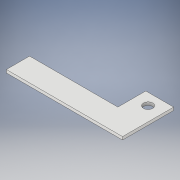
# Autodesk Inventor part: Y-axis X-axis Flag
Saved by Autodesk Inventor 2018 (Build 220112000, 112)
## iProperties
Created: 2013-10-27
Part Number: Y-axis X-axis Flag
Material: Nylon 6/6
Document SubType Name: Modeling
Designer: Gabriel Smolnycki
Mass: 3.40974 g
Surface Area: 15.76 cm^2
Volume: 1.26287 cm^3
Density: 1.13 g/cm^3
Appearance: Smooth - White
Sending System: SolidWorks 2017
Last Author: Gabriel Smolnycki
Last Saved: 2017-09-14
Author: Gabriel Smolnycki
Autodesk Inventor part; units mm, degrees
ref_plane "YZ Plane" through (0, 0, 0) normal (1, 0, 0) x (0, 1, 0)
ref_plane "XZ Plane" through (0, 0, 0) normal (0, 1, 0) x (-1, 0, 0)
ref_plane "XY Plane" through (0, 0, 0) normal (0, 0, 1) x (1, 0, 0)
sketch "Sketch1" plane through (0, 0, 0) normal (0, 1, 0) x (-1, 0, 0)
  line L0 (50, 0) -> (0, 0)
  line L1 (50, -10) -> (50, 0)
  line L2 (12, -10) -> (50, -10)
  line L3 (12, -22) -> (12, -10)
  line L4 (0, -22) -> (12, -22)
  line L5 (0, 0) -> (0, -22)
  constraints: 12 end point, 3 horizontal, 3 vertical, 1 perpendicular
extrude "Extrusion1" add sketch "Sketch1" along normal blind 1.27
sketch "Sketch2" plane through (0, 1.27, 0) normal (0, 1, 0) x (1, 0, 0)
  point P0 (-6, 17)
hole "Hole1" at (-6, 1.27, -17) direction (0, -1, 0) diameter 4 depth 1.27
body "Solid3"
